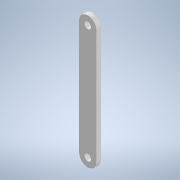
# Autodesk Inventor part: Eslabon_TransPot
Saved by Autodesk Inventor 2022 (Build 260153000, 153)
## iProperties
Created: 2022-02-22
Part Number: Eslabon_TransPot
Material: Generic
Document SubType Name: Modeling
Designer: katha
Density: 1 g/cm^3
Appearance: Default
Author: katha
Autodesk Inventor part; units mm, degrees
ref_plane "YZ Plane" through (0, 0, 0) normal (1, 0, 0) x (0, 1, 0)
ref_plane "XZ Plane" through (0, 0, 0) normal (0, 1, 0) x (-1, 0, 0)
ref_plane "XY Plane" through (0, 0, 0) normal (0, 0, 1) x (1, 0, 0)
sketch "Sketch1" plane through (0, 0, 0) normal (0, 0, 1) x (1, 0, 0)
  circle A0 centre (30, 0) radius 2.3 projected
  circle A1 centre (30, 0) radius 6
  line L0 (24, 0) -> (24, 82)
  line L1 (36, 0) -> (36, 82)
  line L2 (24, 41) -> (36, 41) construction
  circle A2 centre (30, 82) radius 2.3
  circle A3 centre (30, 82) radius 6
  point P0 (0, 0)
  dimension "d0" = 12
  dimension "d1" = 82
  constraints: 6 end point, 3 centre point, 2 coincident, 2 midpoint, 2 point on circle, 2 symmetric about line, 2 tangent, 2 vertical, 1 parallel, 2 other
  measures "d0" diameter of A1
  measures "d1" distance of L0.start L0.end
extrude "Extrusion1" add sketch "Sketch1" along normal blind 3.2
body "Solid1"
